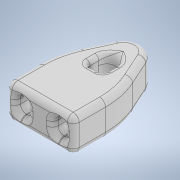
# Autodesk Inventor part: blochek
Saved by Autodesk Inventor 2022 (Build 260153000, 153)
## iProperties
Created: 2023-03-12
Part Number: blochek
Material: Типовые
Document SubType Name: Modeling
Designer: akapu
Density: 1 g/cm^3
Appearance: По умолчанию
Author: akapu
Autodesk Inventor part; units mm, degrees
ref_plane "YZ Plane" through (0, 0, 0) normal (1, 0, 0) x (0, 1, 0)
ref_plane "XZ Plane" through (0, 0, 0) normal (0, 1, 0) x (-1, 0, 0)
ref_plane "XY Plane" through (0, 0, 0) normal (0, 0, 1) x (1, 0, 0)
sketch "Эскиз1" plane through (0, 0, 0) normal (0, 1, 0) x (-1, 0, 0)
  line L0 (4, -6) -> (-4, -6)
  line L1 (-4, -6) -> (-4, 6)
  line L2 (-4, 6) -> (4, 6)
  line L3 (4, 6) -> (4, -6)
  line L4 (4, -6) -> (-4, 6) construction
  line L5 (-4, -6) -> (4, 6) construction
  line L6 (0, -6) -> (0, -4)
  circle A0 centre (0, -4) radius 2
  line L7 (4, 0) -> (1.8229, -4.8229)
  line L8 (-4, 0) -> (-1.8229, -4.8229)
  point P0 (0, 0)
  dimension "d0" = 8
  dimension "d1" = 12
  dimension "d2" = 2
  constraints: 18 end point, 5 midpoint, 3 point on circle, 2 parallel, 2 tangent, 1 centre point, 1 coincident, 1 horizontal, 1 perpendicular, 1 vertical
  measures "d0" distance of L1.end L2.end
  measures "d1" distance of L0.end L1.end
  measures "d2" distance of L6.start L6.end
extrude "Выдавливание1" add sketch "Эскиз1" along normal mid plane 4 contours A0 | L7 A0 L8 L1 L2 L3
sketch "Эскиз2" plane through (0, 0, 0) normal (0, 1, 0) x (-1, 0, 0)
  circle A0 centre (0, 3) radius 1.5
  circle A1 centre (0, 3) radius 3
  line L0 (0, 3) -> (0, 0)
  line L1 (1.5, 3) -> (1.5, 6)
  line L2 (-4, 6) -> (4, 6) projected
  line L3 (3, 3) -> (3, 6)
  line L4 (-3, 3) -> (-3, 6)
  line L5 (-1.5, 3) -> (-1.5, 6)
  dimension "d5" = 3
  dimension "d6" = 6
  dimension "d7" = 3
  constraints: 10 end point, 4 point on circle, 4 point on line, 3 parallel, 3 tangent, 2 centre point, 2 vertical, 1 coincident
  measures "d5" diameter of A0
  measures "d6" diameter of A1
  measures "d7" distance of L0.start L0.end
extrude "Выдавливание2" cut sketch "Эскиз2" along normal mid plane 2 contours L1 A1 L0 A0 | A0 L0 A1 L5 | L1 L2 L3 A1 | A1 L4 L2 L5
fillet "Сопряжение1" radius 0.7 12 edges at (3, -1, 4.5) (-3, -1, 4.5) (0, -1, 0) (0, 1, 0) (3, 1, 4.5) (-3, 1, 4.5) (0, 1, 1.5) (1.5, 1, 4.5) (-1.5, 1, 4.5) (0, -1, 1.5) (1.5, -1, 4.5) (-1.5, -1, 4.5)
fillet "Сопряжение2" radius 0.7 16 edges at (-2.25, -1, 6) (-1.705, -0.795, 6) (-1.5, 0, 6) (-1.705, 0.795, 6) (-2.25, 1, 6) (-2.795, 0.795, 6) (-3, 0, 6) (-2.795, -0.795, 6) (1.705, 0.795, 6) (2.25, 1, 6) (2.795, 0.795, 6) (3, 0, 6) (2.795, -0.795, 6) (2.25, -1, 6) (1.705, -0.795, 6) (1.5, 0, 6)
fillet "Сопряжение3" radius 0.7 14 edges at (0, 2, 6) (4, 2, 3) (-4, 2, 3) (-2.9114, 2, -2.4114) (2.9114, 2, -2.4114) (0, 2, -6) (0, -2, -6) (-2.9114, -2, -2.4114) (2.9114, -2, -2.4114) (4, -2, 3) (4, 0, 6) (-4, -2, 3) (0, -2, 6) (-4, 0, 6)
fillet "Сопряжение4" radius 10 6 edges at (3.795, 1.795, 0.0441) (3.795, -1.795, 0.0441) (4, 0, 0) (-3.795, 1.795, 0.0441) (-3.795, -1.795, 0.0441) (-4, 0, 0)
sketch "Эскиз3" plane through (0, 2, 0) normal (0, 1, 0) x (1, 0, 0)
  arc A0 (1.8229, 4.8229) -> (-1.8229, 4.8229) centre (0, 4) ccw projected
  line L0 (0, 6) -> (0, 3)
  line L1 (0, 3) -> (-1, 3)
  line L2 (-1, 3) -> (1, 3)
  line L3 (1, 3) -> (1, 0.5)
  line L4 (1, 0.5) -> (-1, 0.5)
  line L5 (-1, 0.5) -> (-1, 3)
  point P0 (0, 0)
  dimension "d18" = 3
  dimension "d19" = 2.5
  constraints: 12 end point, 2 horizontal, 2 parallel, 1 perpendicular, 1 point on circle, 1 vertical
  measures "d18" distance of L0.start L0.end
  measures "d19" distance of L2.end L3.end
extrude "Выдавливание3" cut sketch "Эскиз3" against normal blind 4
fillet "Сопряжение6" radius 1 4 edges at (0, 2, -3) (0, -2, -3) (1, 0, -3) (-1, 0, -3)
fillet "Сопряжение7" radius 0.5 16 edges at (0.6659, 2, -3.2435) (1, 2, -1.384) (-0.4384, 2, -3.5388) (-0.8134, 2, -2.9942) (-0.9505, 2, -2.6384) (-1, 2, -1.384) (-1, -2, -1.384) (-0.4384, -2, -3.5388) (-0.8134, -2, -2.9942) (-0.9505, -2, -2.6384) (0.6659, -2, -3.2435) (1, -2, -1.384) (-1, 0, -0.5) (1, 0, -0.5) (0, -2, -0.5) (0, 2, -0.5)
